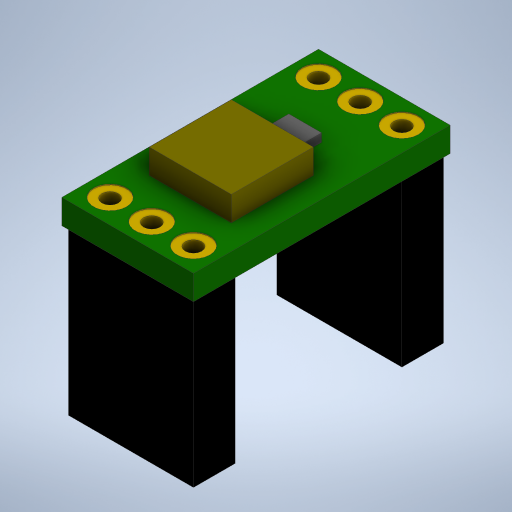
# Autodesk Inventor part: TPS61230A
Saved by Autodesk Inventor 2024.1 (Build 281209000, 209)
## iProperties
Created: 2025-02-20
Part Number: TPS61230A
Material: 一般
Document SubType Name: Modeling
Designer: hibik
Density: 1 g/cm^3
Appearance: 既定
Author: hibik
Autodesk Inventor part; units mm, degrees
ref_plane "YZ Plane" through (0, 0, 0) normal (1, 0, 0) x (0, 1, 0)
ref_plane "XZ Plane" through (0, 0, 0) normal (0, 1, 0) x (-1, 0, 0)
ref_plane "XY Plane" through (0, 0, 0) normal (0, 0, 1) x (1, 0, 0)
sketch "スケッチ1" plane through (0, 0, 0) normal (0, 1, 0) x (-1, 0, 0)
  line L0 (3.81, -5.08) -> (-3.81, -5.08)
  line L1 (-3.81, -5.08) -> (-3.81, -7.62)
  line L2 (-3.81, -7.62) -> (3.81, -7.62)
  line L3 (3.81, -7.62) -> (3.81, -5.08)
  line L4 (3.81, 7.62) -> (-3.81, 7.62)
  line L5 (-3.81, 7.62) -> (-3.81, 5.08)
  line L6 (-3.81, 5.08) -> (3.81, 5.08)
  line L7 (3.81, 5.08) -> (3.81, 7.62)
  line L8 (5.334, 0) -> (-5.334, 0) projected
  point P0 (0, 0)
  point P1 (0, 7.62)
  point P2 (3.81, 6.35)
  point P3 (3.81, -6.35)
  point P4 (-5.334, 0)
  dimension "d0" = 7.62
  dimension "d1" = 2.54
  dimension "d2" = 12.7
  constraints: 16 end point, 5 parallel, 3 midpoint, 2 equal length, 2 horizontal, 2 perpendicular, 1 collinear, 1 vertical alignment, 1 other
  measures "d0" distance of L0.start L0.end
  measures "d1" distance of L2.end L0.start
  measures "d2" distance of point (3.81, 6.35) point (3.81, -6.35)
extrude "押し出し1" add sketch "スケッチ1" along normal blind 10
sketch "スケッチ2" plane through (0, 10, 0) normal (0, 1, 0) x (1, 0, 0)
  line L0 (-4.01, -7.82) -> (4.01, -7.82)
  line L1 (4.01, -7.82) -> (4.01, 7.82)
  line L2 (4.01, 7.82) -> (-4.01, 7.82)
  line L3 (-4.01, 7.82) -> (-4.01, -7.82)
  line L4 (-3.81, -5.08) -> (-3.81, -7.62) projected
  line L5 (-3.81, -7.62) -> (3.81, -7.62) projected
  point P0 (0, 0)
  point P1 (0, -7.82)
  point P2 (-4.01, 0)
  dimension "d7" = 0.2
  dimension "d8" = 0.2
  constraints: 8 end point, 2 midpoint, 2 parallel, 1 horizontal, 1 horizontal alignment, 1 perpendicular, 1 vertical alignment
  measures "d7" distance between parallel lines of L3 L4
  measures "d8" distance between parallel lines of L0 L5
extrude "押し出し2" add sketch "スケッチ2" along normal blind 1.5
sketch "スケッチ3" plane through (0, 11.5, 0) normal (0, 1, 0) x (1, 0, 0)
  line L0 (3.81, -7.62) -> (3.81, -5.08) projected
  line L1 (-3.81, -7.62) -> (3.81, -7.62) projected
  line L2 (-3.81, -5.08) -> (-3.81, -7.62) projected
  line L3 (3.81, -5.08) -> (-3.81, -5.08) projected
  line L4 (3.81, 5.08) -> (3.81, 7.62) projected
  line L5 (-3.81, 5.08) -> (3.81, 5.08) projected
  line L6 (-3.81, 7.62) -> (-3.81, 5.08) projected
  line L7 (3.81, 7.62) -> (-3.81, 7.62) projected
  circle A0 centre (-2.54, -6.35) radius 1
  line L8 (-3.81, -5.08) -> (-3.81, -7.62) projected
  circle A1 centre (0, -6.35) radius 1
  circle A2 centre (2.54, -6.35) radius 1
  line L9 (-5.614, 0) -> (5.614, 0) projected
  circle A3 centre (-2.54, 6.35) radius 1
  line L10 (-3.81, 5.08) -> (-3.81, 7.62)
  circle A4 centre (0, 6.35) radius 1
  circle A5 centre (2.54, 6.35) radius 1
  circle A6 centre (-2.54, -6.35) radius 0.5
  circle A7 centre (0, -6.35) radius 0.5
  circle A8 centre (2.54, -6.35) radius 0.5
  circle A9 centre (-2.54, 6.35) radius 0.5
  circle A10 centre (0, 6.35) radius 0.5
  circle A11 centre (2.54, 6.35) radius 0.5
  line L11 (-2.5, -4) -> (2.5, -4)
  line L12 (2.5, -4) -> (2.5, 1)
  line L13 (2.5, 1) -> (-2.5, 1)
  line L14 (-2.5, 1) -> (-2.5, -4)
  line L15 (-1, 1) -> (1, 1)
  line L16 (1, 1) -> (1, 3)
  line L17 (1, 3) -> (-1, 3)
  line L18 (-1, 3) -> (-1, 1)
  point P0 (0.6683, -5.6061)
  point P1 (-3.81, -6.35)
  point P2 (-3.81, -6.35)
  point P3 (0, 0)
  point P4 (0.6683, 5.6061)
  point P5 (-3.81, 6.35)
  point P6 (-3.81, 6.35)
  point P7 (0, 1)
  point P8 (0, 3)
  dimension "d9" = 2
  dimension "d10" = 2.54
  dimension "d11" = 2.54
  dimension "d12" = 1
  dimension "d13" = 1
  dimension "d14" = 1
  dimension "d15" = 1
  dimension "d16" = 1
  dimension "d17" = 1
  dimension "d18" = 1
  dimension "d19" = 5
  dimension "d20" = 5
  dimension "d21" = 2
  constraints: 18 end point, 10 centre point, 6 symmetric about line, 5 coincident, 4 horizontal alignment, 4 midpoint, 4 parallel, 3 horizontal, 3 perpendicular, 3 vertical alignment, 1 concentric, 1 equal radius, 1 point on line, 9 other
  measures "d9" diameter of A0
  measures "d10" distance of A0.centre point (0, -6.35)
  measures "d11" distance of A2.centre point (0, -6.35)
  measures "d12" diameter of A6
  measures "d13" diameter of A7
  measures "d14" diameter of A8
  measures "d15" diameter of A9
  measures "d16" diameter of A10
  measures "d17" diameter of A11
  measures "d18" distance between parallel lines of L9 L13
  measures "d19" distance of L13.end L11.start
  measures "d20" distance of L11.start L11.end
  measures "d21" distance of L16.end L17.end
extrude "押し出し3" cut sketch "スケッチ3" against normal through all contours A6 | A7 | A8 | A9 | A10 | A11
extrude "押し出し4" cut sketch "スケッチ3" against normal blind 0.05 contours A0 | A1 | A2 | A3 | A4 | A5
extrude "押し出し5" add sketch "スケッチ3" along normal blind 1.5 contours L14 L13 L12 L9 | L9 L12 L11 L14
extrude "押し出し6" add sketch "スケッチ3" along normal blind 0.5 contours L18 L17 L16 L13
equation "\"d11\" = d10"
